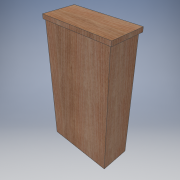
# Autodesk Inventor part: FrenteGrande
Saved by Autodesk Inventor 2016 (Build 200138000, 138)
## iProperties
Created: 2018-06-25
Part Number: FrenteGrande
Material: Wood (Birch)
Document SubType Name: Modeling
Designer: damia
Density: 0.55 g/cm^3
Appearance: Birch - Natural Polished
Mass: 3171.77 g
Surface Area: 8434.79 cm^2
Volume: 5766.85 cm^3
Author: damia
Autodesk Inventor part; units mm, degrees
ref_plane "YZ Plane" through (0, 0, 0) normal (1, 0, 0) x (0, 1, 0)
ref_plane "XZ Plane" through (0, 0, 0) normal (0, 1, 0) x (-1, 0, 0)
ref_plane "XY Plane" through (0, 0, 0) normal (0, 0, 1) x (1, 0, 0)
sketch "Sketch5" plane through (0, 0, 0) normal (0, 0, 1) x (1, 0, 0)
  line L0 (0, 0) -> (370, 0)
  line L1 (370, 0) -> (370, 150)
  line L2 (370, 150) -> (0, 150)
  line L3 (0, 150) -> (0, 0)
  dimension "d15" = 370
  dimension "d16" = 150
  constraints: 8 end point, 2 parallel, 1 horizontal, 1 perpendicular
  measures "d15" distance of L2.end L1.end
  measures "d16" distance of L0.end L1.end
extrude "Extrusion5" add sketch "Sketch5" along normal blind 18
sketch "Sketch6" plane through (0, 0, 0) normal (0, 0, -1) x (-1, 0, 0)
  line L0 (-362.3, 140) -> (-344.3, 140)
  line L1 (-344.3, 140) -> (-344.3, 5)
  line L2 (-344.3, 5) -> (-362.3, 5)
  line L3 (-362.3, 5) -> (-362.3, 140)
  line L4 (-370, 0) -> (-370, 150) projected
  line L5 (0, 0) -> (-370, 0) projected
  line L6 (-25.7, 140) -> (-7.7, 140)
  line L7 (-7.7, 140) -> (-7.7, 5)
  line L8 (-7.7, 5) -> (-25.7, 5)
  line L9 (-25.7, 5) -> (-25.7, 140)
  line L10 (0, 150) -> (0, 0) projected
  dimension "d19" = 18
  dimension "d20" = 135
  dimension "d21" = 7.7
  dimension "d22" = 5
  dimension "d23" = 18
  dimension "d24" = 7.7
  dimension "d25" = 5
  constraints: 16 end point, 4 parallel, 2 horizontal, 2 perpendicular, 1 horizontal alignment
  measures "d19" distance of L1.end L2.end
  measures "d20" distance of L0.end L1.end
  measures "d21" distance between parallel lines of L4 L3
  measures "d22" distance between parallel lines of L5 L2
  measures "d23" distance of L7.end L8.end
  measures "d24" distance between parallel lines of L10 L7
  measures "d25" distance between parallel lines of L5 L8
extrude "Extrusion6" add sketch "Sketch6" along normal blind 550
sketch "Sketch7" plane through (0, 0, -550) normal (0, 0, -1) x (-1, 0, 0)
  line L0 (-344.3, 140) -> (-344.3, 5) projected
  line L1 (-25.7, 5) -> (-25.7, 140) projected
  line L2 (-344.3, 140) -> (-25.7, 140)
  line L3 (-25.7, 140) -> (-25.7, 5)
  line L4 (-25.7, 5) -> (-344.3, 5)
  line L5 (-344.3, 5) -> (-344.3, 140)
  point P0 (0, 0)
  constraints: 8 end point, 2 parallel, 1 horizontal, 1 perpendicular
extrude "Extrusion7" add sketch "Sketch7" against normal blind 18
sketch "Sketch8" plane through (7.7, 5, -550) normal (0, -1, 0) x (1, 0, 0)
  line L0 (354.6, 550) -> (336.6, 550) projected
  line L1 (354.6, 550) -> (354.6, 0) projected
  line L2 (0, 0) -> (354.6, 0) projected
  line L3 (0, 550) -> (0, 0) projected
  line L4 (18, 550) -> (0, 550) projected
  line L5 (18, 550) -> (18, 18) projected
  line L6 (336.6, 18) -> (18, 18) projected
  line L7 (336.6, 550) -> (336.6, 18) projected
  line L8 (362.3, 550) -> (-7.7, 550) projected
extrude "Extrusion8" add sketch "Sketch8" against normal blind 9 contours L7 L6 L5 L8
equation "\"d16\" = Cajon02Altura"
equation "\"d24\" = d21"
equation "\"d25\" = d22"
equation "\"Cajon02Altura\" = 150"
body "Solid2"
